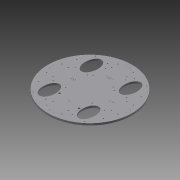
# Autodesk Inventor part: Base_Acryllic
Saved by Autodesk Inventor 2016 (Build 200138000, 138)
## iProperties
Created: 2016-03-29
Part Number: Base_Acryllic
Material: Generic
Document SubType Name: Modeling
Designer: Ethan
Density: 1 g/cm^3
Appearance: Default
Author: Ethan
Autodesk Inventor part; units mm, degrees
(part 1 of 2)
ref_plane "YZ Plane" through (0, 0, 0) normal (1, 0, 0) x (0, 1, 0)
ref_plane "XZ Plane" through (0, 0, 0) normal (0, 1, 0) x (-1, 0, 0)
ref_plane "XY Plane" through (0, 0, 0) normal (0, 0, 1) x (1, 0, 0)
sketch "Sketch1" plane through (0, 0, 0) normal (0, 1, 0) x (-1, 0, 0)
  circle A0 centre (0, 0) radius 139.7
  circle A1 centre (-118.5333, 25.4) radius 1.5875
  circle A2 centre (-97.3667, 25.4) radius 1.5875
  circle A3 centre (-118.5333, -25.4) radius 1.5875
  circle A4 centre (-97.3667, -25.4) radius 1.5875
  ellipse E0 centre (-65.0875, 69.8532) end of major axis (-65.0875, 36.5157) minor radius 20.6375
  ellipse E1 centre (-65.0875, -69.8532) end of major axis (-65.0875, -36.5157) minor radius 20.6375
  ellipse E2 centre (65.0875, 69.8532) end of major axis (65.0875, 36.5157) minor radius 20.6375
  ellipse E3 centre (65.0875, -69.8532) end of major axis (65.0875, -36.5157) minor radius 20.6375
  circle A5 centre (-38.1, 74.0494) radius 3.175
  circle A6 centre (38.1, 62.9369) radius 3.175
  circle A7 centre (85.725, 103.1907) radius 1.5875
  circle A8 centre (44.45, 103.1907) radius 1.5875
  circle A9 centre (85.725, 36.5157) radius 1.5875
  circle A10 centre (44.45, 36.5157) radius 1.5875
  circle A11 centre (44.45, -36.5157) radius 1.5875
  circle A12 centre (44.45, -103.1907) radius 1.5875
  circle A13 centre (85.725, -103.1907) radius 1.5875
  circle A14 centre (85.725, -36.5157) radius 1.5875
  circle A15 centre (33.3375, -43.706) radius 1.5875
  circle A16 centre (33.3375, -84.981) radius 1.5875
  circle A17 centre (-33.3375, -84.981) radius 1.5875
  circle A18 centre (-33.3375, -43.706) radius 1.5875
  circle A19 centre (-44.45, 36.5157) radius 1.5875
  circle A20 centre (-44.45, 103.1907) radius 1.5875
  circle A21 centre (-85.725, 103.1907) radius 1.5875
  circle A22 centre (-85.725, 36.5157) radius 1.5875
  circle A23 centre (-85.725, -36.5157) radius 1.5875
  circle A24 centre (-44.45, -36.5157) radius 1.5875
  circle A25 centre (-44.45, -103.1907) radius 1.5875
  circle A26 centre (-85.725, -103.1907) radius 1.5875
  circle A27 centre (-25.4, -118.5333) radius 1.5875
  circle A28 centre (-25.4, -97.3667) radius 1.5875
  circle A29 centre (25.4, -97.3667) radius 1.5875
  circle A30 centre (25.4, -118.5333) radius 1.5875
  circle A31 centre (118.5333, -25.4) radius 1.5875
  circle A32 centre (97.3667, -25.4) radius 1.5875
  circle A33 centre (97.3667, 25.4) radius 1.5875
  circle A34 centre (118.5333, 25.4) radius 1.5875
  circle A35 centre (25.4, 118.5333) radius 1.5875
  circle A36 centre (25.4, 97.3667) radius 1.5875
  circle A37 centre (-25.4, 97.3667) radius 1.5875
  circle A38 centre (-25.4, 118.5333) radius 1.5875
  circle A39 centre (107.2204, 62.9369) radius 1.5875
  circle A40 centre (-107.2204, 62.9369) radius 1.5875
  circle A41 centre (107.2204, -62.9369) radius 1.5875
  circle A42 centre (-107.2204, -62.9369) radius 1.5875
  circle A43 centre (6.25, 127) radius 1.1303
  circle A44 centre (-6.25, 127) radius 1.1303
  circle A45 centre (-127, 6.25) radius 1.1303
  circle A46 centre (-127, -6.25) radius 1.1303
  circle A47 centre (-6.25, -127) radius 1.1303
  circle A48 centre (6.25, -127) radius 1.1303
  circle A49 centre (127, -6.25) radius 1.1303
  circle A50 centre (127, 6.25) radius 1.1303
  line L0 (-37.9059, 73.7607) -> (38.0077, 73.7607) construction
  line L1 (38.0077, 73.7607) -> (38.0077, 62.868) construction
  line L2 (38.0077, 62.868) -> (-37.9059, 62.868) construction
  line L3 (-37.9059, 62.868) -> (-37.9059, 73.7607) construction
  line L4 (-34.0251, -43.002) -> (33.1245, -43.002) construction
  line L5 (33.1245, -43.002) -> (33.1245, -85.2103) construction
  line L6 (33.1245, -85.2103) -> (-34.0251, -85.2103) construction
  line L7 (-34.0251, -85.2103) -> (-34.0251, -43.002) construction
  line L8 (-12.7946, 24.5361) -> (126.9054, 24.5361) construction
  line L9 (126.9054, 24.5361) -> (126.9054, -26.2639) construction
  line L10 (126.9054, -26.2639) -> (-12.7946, -26.2639) construction
  line L11 (-12.7946, -26.2639) -> (-12.7946, 24.5361) construction
  line L12 (-126.5016, 32.6762) -> (-18.5516, 32.6762) construction
  line L13 (-18.5516, 32.6762) -> (-18.5516, -30.8238) construction
  line L14 (-18.5516, -30.8238) -> (-126.5016, -30.8238) construction
  line L15 (-126.5016, -30.8238) -> (-126.5016, 32.6762) construction
  line L16 (-6.9664, 66.7583) -> (-6.9664, 69.2258)
  line L17 (-6.9664, 69.2258) -> (-7.868, 69.2258)
  line L18 (-7.868, 69.2258) -> (-7.868, 69.8063)
  line L19 (-7.868, 69.8063) -> (-5.2991, 69.8063)
  line L20 (-5.2991, 69.8063) -> (-5.2991, 69.2258)
  line L21 (-5.2991, 69.2258) -> (-6.2007, 69.2258)
  line L22 (-6.2007, 69.2258) -> (-6.2007, 66.7583)
  line L23 (-6.2007, 66.7583) -> (-6.9664, 66.7583)
  line L24 (-3.7208, 67.8204) -> (-5.0768, 67.8204)
  line L25 (-5.0768, 67.8204) -> (-5.0768, 68.3885)
  line L26 (-5.0768, 68.3885) -> (-3.7208, 68.3885)
  line L27 (-3.7208, 68.3885) -> (-3.7208, 67.8204)
  spline S0 degree 2 poles (-0.742, 67.6919) (-0.742, 67.4647) (-0.9149, 67.1214) (-1.0581, 67.0078) knots 0 0 0 1 2 2 2
  spline S1 degree 2 poles (-1.0581, 67.0078) (-1.231, 66.8719) (-1.641, 66.7583) (-1.9597, 66.7583) knots 0 0 0 1 2 2 2
  line L28 (-1.9597, 66.7583) -> (-3.1774, 66.7583)
  line L29 (-3.1774, 66.7583) -> (-3.1774, 69.8063)
  line L30 (-3.1774, 69.8063) -> (-2.1029, 69.8063)
  spline S2 degree 2 poles (-2.1029, 69.8063) (-1.767, 69.8063) (-1.4212, 69.7544) (-1.2705, 69.6729) knots 0 0 0 1 2 2 2
  spline S3 degree 2 poles (-1.2705, 69.6729) (-1.1051, 69.5864) (-0.9445, 69.29) (-0.9445, 69.0974) knots 0 0 0 1 2 2 2
  spline S4 degree 2 poles (-0.9445, 69.0974) (-0.9445, 68.8751) (-1.1668, 68.5268) (-1.3644, 68.4453) knots 0 0 0 1 2 2 2
  line L31 (-1.3644, 68.4453) -> (-1.3644, 68.4305)
  spline S5 degree 2 poles (-1.3644, 68.4305) (-1.0804, 68.3712) (-0.742, 68.0032) (-0.742, 67.6919) knots 0 0 0 1 2 2 2
  spline S6 degree 2 poles (-1.5324, 67.7043) (-1.5324, 67.8476) (-1.646, 68.0081) (-1.7596, 68.0501) knots 0 0 0 1 2 2 2
  spline S7 degree 2 poles (-1.7596, 68.0501) (-1.8288, 68.0773) (-2.0733, 68.0822) (-2.2758, 68.0822) knots 0 0 0 1 2 2 2
  line L32 (-2.2758, 68.0822) -> (-2.4166, 68.0822)
  line L33 (-2.4166, 68.0822) -> (-2.4166, 67.314)
  line L34 (-2.4166, 67.314) -> (-2.3746, 67.314)
  spline S8 degree 2 poles (-2.3746, 67.314) (-2.0782, 67.314) (-1.851, 67.3214) (-1.7324, 67.3733) knots 0 0 0 1 2 2 2
  spline S9 degree 2 poles (-1.7324, 67.3733) (-1.6287, 67.4202) (-1.5324, 67.5931) (-1.5324, 67.7043) knots 0 0 0 1 2 2 2
  spline S10 degree 2 poles (-1.7226, 68.9467) (-1.7226, 69.0208) (-1.7991, 69.1764) (-1.8782, 69.211) knots 0 0 0 1 2 2 2
  spline S11 degree 2 poles (-1.8782, 69.211) (-1.9523, 69.2456) (-2.1598, 69.2505) (-2.3648, 69.2505) knots 0 0 0 1 2 2 2
  line L35 (-2.3648, 69.2505) -> (-2.4166, 69.2505)
  line L36 (-2.4166, 69.2505) -> (-2.4166, 68.6034)
  line L37 (-2.4166, 68.6034) -> (-2.3203, 68.6034)
  spline S12 degree 2 poles (-2.3203, 68.6034) (-2.1252, 68.6034) (-1.9671, 68.6108) (-1.8831, 68.6503) knots 0 0 0 1 2 2 2
  spline S13 degree 2 poles (-1.8831, 68.6503) (-1.7917, 68.6948) (-1.7226, 68.8454) (-1.7226, 68.9467) knots 0 0 0 1 2 2 2
  line L38 (0.372, 66.7583) -> (-0.3443, 66.7583)
  line L39 (-0.3443, 66.7583) -> (-0.3443, 69.9421)
  line L40 (-0.3443, 69.9421) -> (0.372, 69.9421)
  line L41 (0.372, 69.9421) -> (0.372, 66.7583)
  spline S14 degree 2 poles (3.1261, 67.9068) (3.1261, 67.3387) (2.5061, 66.6866) (1.9405, 66.6866) knots 0 0 0 1 2 2 2
  spline S15 degree 2 poles (1.9405, 66.6866) (1.3773, 66.6866) (0.7524, 67.3387) (0.7524, 67.9068) knots 0 0 0 1 2 2 2
  spline S16 degree 2 poles (0.7524, 67.9068) (0.7524, 68.4799) (1.3773, 69.1295) (1.9405, 69.1295) knots 0 0 0 1 2 2 2
  spline S17 degree 2 poles (1.9405, 69.1295) (2.5036, 69.1295) (3.1261, 68.4774) (3.1261, 67.9068) knots 0 0 0 1 2 2 2
  spline S18 degree 2 poles (2.3925, 67.9019) (2.3925, 68.1069) (2.3258, 68.3811) (2.2665, 68.4626) knots 0 0 0 1 2 2 2
  spline S19 degree 2 poles (2.2665, 68.4626) (2.2023, 68.549) (2.0417, 68.6157) (1.9405, 68.6157) knots 0 0 0 1 2 2 2
  spline S20 degree 2 poles (1.9405, 68.6157) (1.8417, 68.6157) (1.6861, 68.5565) (1.6218, 68.4725) knots 0 0 0 1 2 2 2
  spline S21 degree 2 poles (1.6218, 68.4725) (1.5601, 68.3934) (1.486, 68.1143) (1.486, 67.9019) knots 0 0 0 1 2 2 2
  spline S22 degree 2 poles (1.486, 67.9019) (1.486, 67.6919) (1.5552, 67.4326) (1.612, 67.3536) knots 0 0 0 1 2 2 2
  spline S23 degree 2 poles (1.612, 67.3536) (1.6688, 67.2745) (1.8417, 67.2004) (1.9454, 67.2004) knots 0 0 0 1 2 2 2
  spline S24 degree 2 poles (1.9454, 67.2004) (2.0319, 67.2004) (2.2097, 67.2745) (2.264, 67.3486) knots 0 0 0 1 2 2 2
  spline S25 degree 2 poles (2.264, 67.3486) (2.3258, 67.4351) (2.3925, 67.6845) (2.3925, 67.9019) knots 0 0 0 1 2 2 2
  spline S26 degree 2 poles (4.6328, 66.6965) (4.3487, 66.6965) (3.877, 66.8398) (3.7016, 66.988) knots 0 0 0 1 2 2 2
  spline S27 degree 2 poles (3.7016, 66.988) (3.5312, 67.1387) (3.3385, 67.5907) (3.3385, 67.897) knots 0 0 0 1 2 2 2
  spline S28 degree 2 poles (3.3385, 67.897) (3.3385, 68.2279) (3.546, 68.6898) (3.7263, 68.838) knots 0 0 0 1 2 2 2
  spline S29 degree 2 poles (3.7263, 68.838) (3.8967, 68.9813) (4.3611, 69.1196) (4.613, 69.1196) knots 0 0 0 1 2 2 2
  spline S30 degree 2 poles (4.613, 69.1196) (4.8032, 69.1196) (5.1836, 69.0307) (5.3763, 68.9344) knots 0 0 0 1 2 2 2
  line L42 (5.3763, 68.9344) -> (5.3763, 68.3218)
  line L43 (5.3763, 68.3218) -> (5.2849, 68.3218)
  spline S31 degree 2 poles (5.2849, 68.3218) (5.2404, 68.3638) (5.1169, 68.4626) (5.0428, 68.5021) knots 0 0 0 1 2 2 2
  spline S32 degree 2 poles (5.0428, 68.5021) (4.9638, 68.5466) (4.7686, 68.6059) (4.6476, 68.6059) knots 0 0 0 1 2 2 2
  spline S33 degree 2 poles (4.6476, 68.6059) (4.3734, 68.6059) (4.0721, 68.223) (4.0721, 67.897) knots 0 0 0 1 2 2 2
  spline S34 degree 2 poles (4.0721, 67.897) (4.0721, 67.5512) (4.3932, 67.2103) (4.66, 67.2103) knots 0 0 0 1 2 2 2
  spline S35 degree 2 poles (4.66, 67.2103) (4.7958, 67.2103) (4.9984, 67.272) (5.0725, 67.3165) knots 0 0 0 1 2 2 2
  spline S36 degree 2 poles (5.0725, 67.3165) (5.1441, 67.3585) (5.2478, 67.4524) (5.2849, 67.4894) knots 0 0 0 1 2 2 2
  line L44 (5.2849, 67.4894) -> (5.3763, 67.4894)
  line L45 (5.3763, 67.4894) -> (5.3763, 66.8744)
  spline S37 degree 2 poles (5.3763, 66.8744) (5.3145, 66.8472) (5.154, 66.778) (5.07, 66.7558) knots 0 0 0 1 2 2 2
  spline S38 degree 2 poles (5.07, 66.7558) (4.9662, 66.7262) (4.7835, 66.6965) (4.6328, 66.6965) knots 0 0 0 1 2 2 2
  line L46 (8.0192, 66.7583) -> (7.167, 66.7583)
  line L47 (7.167, 66.7583) -> (6.5446, 67.7562)
  line L48 (6.5446, 67.7562) -> (6.4334, 67.608)
  line L49 (6.4334, 67.608) -> (6.4334, 66.7583)
  line L50 (6.4334, 66.7583) -> (5.7171, 66.7583)
  line L51 (5.7171, 66.7583) -> (5.7171, 69.9421)
  line L52 (5.7171, 69.9421) -> (6.4334, 69.9421)
  line L53 (6.4334, 69.9421) -> (6.4334, 68.1588)
  line L54 (6.4334, 68.1588) -> (7.1127, 69.0579)
  line L55 (7.1127, 69.0579) -> (7.9599, 69.0579)
  line L56 (7.9599, 69.0579) -> (7.1547, 68.0674)
  line L57 (7.1547, 68.0674) -> (8.0192, 66.7583)
  line L58 (51.3892, 2.9174) -> (50.0875, 0.4746)
  line L59 (50.0875, 0.4746) -> (49.2378, 0.4746)
  line L60 (49.2378, 0.4746) -> (50.5987, 2.947)
  line L61 (50.5987, 2.947) -> (49.1464, 2.947)
  line L62 (49.1464, 2.947) -> (49.1464, 3.5226)
  line L63 (49.1464, 3.5226) -> (51.3892, 3.5226)
  line L64 (51.3892, 3.5226) -> (51.3892, 2.9174)
  line L65 (52.5921, 0.4746) -> (51.8683, 0.4746)
  line L66 (51.8683, 0.4746) -> (51.8683, 1.2798)
  line L67 (51.8683, 1.2798) -> (52.5921, 1.2798)
  line L68 (52.5921, 1.2798) -> (52.5921, 0.4746)
  line L69 (55.435, 0.4746) -> (53.1947, 0.4746)
  line L70 (53.1947, 0.4746) -> (53.1947, 0.971)
  spline S39 degree 2 poles (53.1947, 0.971) (53.4788, 1.1983) (53.9333, 1.5984) (54.1037, 1.7787) knots 0 0 0 1 2 2 2
  spline S40 degree 2 poles (54.1037, 1.7787) (54.3285, 2.0134) (54.5285, 2.3715) (54.5285, 2.5592) knots 0 0 0 1 2 2 2
  spline S41 degree 2 poles (54.5285, 2.5592) (54.5285, 2.7717) (54.2741, 2.9989) (54.0469, 2.9989) knots 0 0 0 1 2 2 2
  spline S42 degree 2 poles (54.0469, 2.9989) (53.9308, 2.9989) (53.7233, 2.9421) (53.6171, 2.8976) knots 0 0 0 1 2 2 2
  spline S43 degree 2 poles (53.6171, 2.8976) (53.5134, 2.8507) (53.3652, 2.7519) (53.3281, 2.7272) knots 0 0 0 1 2 2 2
  line L71 (53.3281, 2.7272) -> (53.2688, 2.7272)
  line L72 (53.2688, 2.7272) -> (53.2688, 3.3916)
  spline S44 degree 2 poles (53.2688, 3.3916) (53.3973, 3.4534) (53.9456, 3.5818) (54.2, 3.5818) knots 0 0 0 1 2 2 2
  spline S45 degree 2 poles (54.2, 3.5818) (54.7434, 3.5818) (55.3017, 3.0977) (55.3017, 2.6605) knots 0 0 0 1 2 2 2
  spline S46 degree 2 poles (55.3017, 2.6605) (55.3017, 2.3913) (55.0472, 1.8726) (54.7533, 1.5762) knots 0 0 0 1 2 2 2
  spline S47 degree 2 poles (54.7533, 1.5762) (54.5681, 1.3934) (54.2198, 1.1093) (54.1432, 1.0501) knots 0 0 0 1 2 2 2
  line L73 (54.1432, 1.0501) -> (55.435, 1.0501)
  line L74 (55.435, 1.0501) -> (55.435, 0.4746)
  line L75 (59.6439, 3.5226) -> (58.5967, 0.4746)
  line L76 (58.5967, 0.4746) -> (57.7988, 0.4746)
  line L77 (57.7988, 0.4746) -> (56.7516, 3.5226)
  line L78 (56.7516, 3.5226) -> (57.5444, 3.5226)
  line L79 (57.5444, 3.5226) -> (58.2089, 1.4551)
  line L80 (58.2089, 1.4551) -> (58.8708, 3.5226)
  line L81 (58.8708, 3.5226) -> (59.6439, 3.5226)
  spline S48 degree 2 poles (62.0917, 1.6231) (62.0917, 1.055) (61.4718, 0.4029) (60.9061, 0.4029) knots 0 0 0 1 2 2 2
  spline S49 degree 2 poles (60.9061, 0.4029) (60.343, 0.4029) (59.718, 1.055) (59.718, 1.6231) knots 0 0 0 1 2 2 2
  spline S50 degree 2 poles (59.718, 1.6231) (59.718, 2.1962) (60.343, 2.8458) (60.9061, 2.8458) knots 0 0 0 1 2 2 2
  spline S51 degree 2 poles (60.9061, 2.8458) (61.4693, 2.8458) (62.0917, 2.1937) (62.0917, 1.6231) knots 0 0 0 1 2 2 2
  spline S52 degree 2 poles (61.3581, 1.6182) (61.3581, 1.8232) (61.2914, 2.0974) (61.2322, 2.1789) knots 0 0 0 1 2 2 2
  spline S53 degree 2 poles (61.2322, 2.1789) (61.1679, 2.2653) (61.0074, 2.332) (60.9061, 2.332) knots 0 0 0 1 2 2 2
  spline S54 degree 2 poles (60.9061, 2.332) (60.8073, 2.332) (60.6517, 2.2727) (60.5875, 2.1887) knots 0 0 0 1 2 2 2
  spline S55 degree 2 poles (60.5875, 2.1887) (60.5257, 2.1097) (60.4516, 1.8306) (60.4516, 1.6182) knots 0 0 0 1 2 2 2
  spline S56 degree 2 poles (60.4516, 1.6182) (60.4516, 1.4082) (60.5208, 1.1489) (60.5776, 1.0698) knots 0 0 0 1 2 2 2
  spline S57 degree 2 poles (60.5776, 1.0698) (60.6344, 0.9908) (60.8073, 0.9167) (60.9111, 0.9167) knots 0 0 0 1 2 2 2
  spline S58 degree 2 poles (60.9111, 0.9167) (60.9975, 0.9167) (61.1754, 0.9908) (61.2297, 1.0649) knots 0 0 0 1 2 2 2
  spline S59 degree 2 poles (61.2297, 1.0649) (61.2914, 1.1513) (61.3581, 1.4008) (61.3581, 1.6182) knots 0 0 0 1 2 2 2
  line L82 (63.1884, 0.4746) -> (62.4721, 0.4746)
  line L83 (62.4721, 0.4746) -> (62.4721, 3.6584)
  line L84 (62.4721, 3.6584) -> (63.1884, 3.6584)
  line L85 (63.1884, 3.6584) -> (63.1884, 0.4746)
  spline S60 degree 2 poles (64.6161, 0.4301) (64.1789, 0.4301) (63.7788, 0.7907) (63.7788, 1.2007) knots 0 0 0 1 2 2 2
  line L86 (63.7788, 1.2007) -> (63.7788, 2.2752)
  line L87 (63.7788, 2.2752) -> (63.5046, 2.2752)
  line L88 (63.5046, 2.2752) -> (63.5046, 2.7741)
  line L89 (63.5046, 2.7741) -> (63.7788, 2.7741)
  line L90 (63.7788, 2.7741) -> (63.7788, 3.4312)
  line L91 (63.7788, 3.4312) -> (64.4951, 3.4312)
  line L92 (64.4951, 3.4312) -> (64.4951, 2.7741)
  line L93 (64.4951, 2.7741) -> (65.1867, 2.7741)
  line L94 (65.1867, 2.7741) -> (65.1867, 2.2752)
  line L95 (65.1867, 2.2752) -> (64.4951, 2.2752)
  line L96 (64.4951, 2.2752) -> (64.4951, 1.4576)
  spline S61 degree 2 poles (64.4951, 1.4576) (64.4951, 1.3366) (64.5, 1.1563) (64.5296, 1.0846) knots 0 0 0 1 2 2 2
  spline S62 degree 2 poles (64.5296, 1.0846) (64.5593, 1.013) (64.705, 0.929) (64.8433, 0.929) knots 0 0 0 1 2 2 2
  spline S63 degree 2 poles (64.8433, 0.929) (64.9026, 0.929) (65.0879, 0.9784) (65.1249, 0.9982) knots 0 0 0 1 2 2 2
  line L97 (65.1249, 0.9982) -> (65.1867, 0.9982)
  line L98 (65.1867, 0.9982) -> (65.1867, 0.4943)
  spline S64 degree 2 poles (65.1867, 0.4943) (65.0706, 0.4647) (64.8088, 0.4301) (64.6161, 0.4301) knots 0 0 0 1 2 2 2
  spline S65 degree 2 poles (52.0079, -3.6102) (52.0079, -3.8375) (51.835, -4.1808) (51.6917, -4.2944) knots 0 0 0 1 2 2 2
  spline S66 degree 2 poles (51.6917, -4.2944) (51.5188, -4.4303) (51.1088, -4.5439) (50.7902, -4.5439) knots 0 0 0 1 2 2 2
  line L99 (50.7902, -4.5439) -> (49.5725, -4.5439)
  line L100 (49.5725, -4.5439) -> (49.5725, -1.4959)
  line L101 (49.5725, -1.4959) -> (50.6469, -1.4959)
  spline S67 degree 2 poles (50.6469, -1.4959) (50.9828, -1.4959) (51.3286, -1.5478) (51.4793, -1.6293) knots 0 0 0 1 2 2 2
  spline S68 degree 2 poles (51.4793, -1.6293) (51.6448, -1.7157) (51.8054, -2.0121) (51.8054, -2.2048) knots 0 0 0 1 2 2 2
  spline S69 degree 2 poles (51.8054, -2.2048) (51.8054, -2.4271) (51.583, -2.7754) (51.3854, -2.8569) knots 0 0 0 1 2 2 2
  line L102 (51.3854, -2.8569) -> (51.3854, -2.8717)
  spline S70 degree 2 poles (51.3854, -2.8717) (51.6695, -2.931) (52.0079, -3.299) (52.0079, -3.6102) knots 0 0 0 1 2 2 2
  spline S71 degree 2 poles (51.2175, -3.5979) (51.2175, -3.4546) (51.1039, -3.2941) (50.9902, -3.2521) knots 0 0 0 1 2 2 2
  spline S72 degree 2 poles (50.9902, -3.2521) (50.9211, -3.2249) (50.6766, -3.22) (50.474, -3.22) knots 0 0 0 1 2 2 2
  line L103 (50.474, -3.22) -> (50.3332, -3.22)
  line L104 (50.3332, -3.22) -> (50.3332, -3.9881)
  line L105 (50.3332, -3.9881) -> (50.3752, -3.9881)
  spline S73 degree 2 poles (50.3752, -3.9881) (50.6716, -3.9881) (50.8989, -3.9807) (51.0174, -3.9289) knots 0 0 0 1 2 2 2
  spline S74 degree 2 poles (51.0174, -3.9289) (51.1212, -3.8819) (51.2175, -3.709) (51.2175, -3.5979) knots 0 0 0 1 2 2 2
  spline S75 degree 2 poles (51.0273, -2.3555) (51.0273, -2.2814) (50.9507, -2.1258) (50.8717, -2.0912) knots 0 0 0 1 2 2 2
  spline S76 degree 2 poles (50.8717, -2.0912) (50.7976, -2.0566) (50.5901, -2.0517) (50.3851, -2.0517) knots 0 0 0 1 2 2 2
  line L106 (50.3851, -2.0517) -> (50.3332, -2.0517)
  line L107 (50.3332, -2.0517) -> (50.3332, -2.6988)
  line L108 (50.3332, -2.6988) -> (50.4296, -2.6988)
  spline S77 degree 2 poles (50.4296, -2.6988) (50.6247, -2.6988) (50.7828, -2.6914) (50.8667, -2.6519) knots 0 0 0 1 2 2 2
  spline S78 degree 2 poles (50.8667, -2.6519) (50.9581, -2.6074) (51.0273, -2.4567) (51.0273, -2.3555) knots 0 0 0 1 2 2 2
  spline S79 degree 2 poles (53.6727, -4.2994) (53.5986, -4.3611) (53.4825, -4.4599) (53.3837, -4.5093) knots 0 0 0 1 2 2 2
  spline S80 degree 2 poles (53.3837, -4.5093) (53.2874, -4.5563) (53.1046, -4.6057) (52.9416, -4.6057) knots 0 0 0 1 2 2 2
  spline S81 degree 2 poles (52.9416, -4.6057) (52.6353, -4.6057) (52.2327, -4.1956) (52.2327, -3.8844) knots 0 0 0 1 2 2 2
  spline S82 degree 2 poles (52.2327, -3.8844) (52.2327, -3.63) (52.4377, -3.3138) (52.6303, -3.2224) knots 0 0 0 1 2 2 2
  spline S83 degree 2 poles (52.6303, -3.2224) (52.8255, -3.1286) (53.3664, -3.0545) (53.6776, -3.0347) knots 0 0 0 1 2 2 2
  line L109 (53.6776, -3.0347) -> (53.6776, -3.0224)
  spline S84 degree 2 poles (53.6776, -3.0224) (53.6776, -2.8322) (53.396, -2.6864) (53.1145, -2.6864) knots 0 0 0 1 2 2 2
  spline S85 degree 2 poles (53.1145, -2.6864) (52.9885, -2.6864) (52.6476, -2.7778) (52.4871, -2.8495) knots 0 0 0 1 2 2 2
  line L110 (52.4871, -2.8495) -> (52.4253, -2.8495)
  line L111 (52.4253, -2.8495) -> (52.4253, -2.2937)
  spline S86 degree 2 poles (52.4253, -2.2937) (52.5315, -2.2641) (53.0058, -2.1801) (53.2478, -2.1801) knots 0 0 0 1 2 2 2
  spline S87 degree 2 poles (53.2478, -2.1801) (53.8406, -2.1801) (54.384, -2.5753) (54.384, -2.9804) knots 0 0 0 1 2 2 2
  line L112 (54.384, -2.9804) -> (54.384, -4.5439)
  line L113 (54.384, -4.5439) -> (53.6727, -4.5439)
  line L114 (53.6727, -4.5439) -> (53.6727, -4.2994)
  line L115 (53.6727, -3.9437) -> (53.6727, -3.467)
  spline S88 degree 2 poles (53.6727, -3.467) (53.4899, -3.4843) (53.2651, -3.5114) (53.1564, -3.551) knots 0 0 0 1 2 2 2
  spline S89 degree 2 poles (53.1564, -3.551) (53.0601, -3.5831) (52.9564, -3.7164) (52.9564, -3.8251) knots 0 0 0 1 2 2 2
  spline S90 degree 2 poles (52.9564, -3.8251) (52.9564, -3.9857) (53.1317, -4.1067) (53.3022, -4.1067) knots 0 0 0 1 2 2 2
  spline S91 degree 2 poles (53.3022, -4.1067) (53.396, -4.1067) (53.5936, -4.0203) (53.6727, -3.9437) knots 0 0 0 1 2 2 2
  spline S92 degree 2 poles (55.7944, -4.5884) (55.3572, -4.5884) (54.9571, -4.2277) (54.9571, -3.8177) knots 0 0 0 1 2 2 2
  line L116 (54.9571, -3.8177) -> (54.9571, -2.7433)
  line L117 (54.9571, -2.7433) -> (54.6829, -2.7433)
  line L118 (54.6829, -2.7433) -> (54.6829, -2.2443)
  line L119 (54.6829, -2.2443) -> (54.9571, -2.2443)
  line L120 (54.9571, -2.2443) -> (54.9571, -1.5873)
  line L121 (54.9571, -1.5873) -> (55.6734, -1.5873)
  line L122 (55.6734, -1.5873) -> (55.6734, -2.2443)
  line L123 (55.6734, -2.2443) -> (56.365, -2.2443)
  line L124 (56.365, -2.2443) -> (56.365, -2.7433)
  line L125 (56.365, -2.7433) -> (55.6734, -2.7433)
  line L126 (55.6734, -2.7433) -> (55.6734, -3.5608)
  spline S93 degree 2 poles (55.6734, -3.5608) (55.6734, -3.6819) (55.6783, -3.8622) (55.708, -3.9338) knots 0 0 0 1 2 2 2
  spline S94 degree 2 poles (55.708, -3.9338) (55.7376, -4.0054) (55.8833, -4.0894) (56.0217, -4.0894) knots 0 0 0 1 2 2 2
  spline S95 degree 2 poles (56.0217, -4.0894) (56.0809, -4.0894) (56.2662, -4.04) (56.3033, -4.0203) knots 0 0 0 1 2 2 2
  line L127 (56.3033, -4.0203) -> (56.365, -4.0203)
  line L128 (56.365, -4.0203) -> (56.365, -4.5241)
  spline S96 degree 2 poles (56.365, -4.5241) (56.2489, -4.5538) (55.9871, -4.5884) (55.7944, -4.5884) knots 0 0 0 1 2 2 2
  spline S97 degree 2 poles (57.5358, -4.5884) (57.0986, -4.5884) (56.6985, -4.2277) (56.6985, -3.8177) knots 0 0 0 1 2 2 2
  line L129 (56.6985, -3.8177) -> (56.6985, -2.7433)
  line L130 (56.6985, -2.7433) -> (56.4243, -2.7433)
  line L131 (56.4243, -2.7433) -> (56.4243, -2.2443)
  line L132 (56.4243, -2.2443) -> (56.6985, -2.2443)
  line L133 (56.6985, -2.2443) -> (56.6985, -1.5873)
  line L134 (56.6985, -1.5873) -> (57.4148, -1.5873)
  line L135 (57.4148, -1.5873) -> (57.4148, -2.2443)
  line L136 (57.4148, -2.2443) -> (58.1064, -2.2443)
  line L137 (58.1064, -2.2443) -> (58.1064, -2.7433)
  line L138 (58.1064, -2.7433) -> (57.4148, -2.7433)
  line L139 (57.4148, -2.7433) -> (57.4148, -3.5608)
  spline S98 degree 2 poles (57.4148, -3.5608) (57.4148, -3.6819) (57.4197, -3.8622) (57.4493, -3.9338) knots 0 0 0 1 2 2 2
  spline S99 degree 2 poles (57.4493, -3.9338) (57.479, -4.0054) (57.6247, -4.0894) (57.763, -4.0894) knots 0 0 0 1 2 2 2
  spline S100 degree 2 poles (57.763, -4.0894) (57.8223, -4.0894) (58.0076, -4.04) (58.0446, -4.0203) knots 0 0 0 1 2 2 2
  line L140 (58.0446, -4.0203) -> (58.1064, -4.0203)
  line L141 (58.1064, -4.0203) -> (58.1064, -4.5241)
  spline S101 degree 2 poles (58.1064, -4.5241) (57.9903, -4.5538) (57.7284, -4.5884) (57.5358, -4.5884) knots 0 0 0 1 2 2 2
  spline S102 degree 2 poles (59.576, -4.6057) (58.9239, -4.6057) (58.2299, -3.9832) (58.2299, -3.4077) knots 0 0 0 1 2 2 2
  spline S103 degree 2 poles (58.2299, -3.4077) (58.2299, -2.8445) (58.877, -2.1727) (59.4599, -2.1727) knots 0 0 0 1 2 2 2
  spline S104 degree 2 poles (59.4599, -2.1727) (59.986, -2.1727) (60.5196, -2.7433) (60.5196, -3.2718) knots 0 0 0 1 2 2 2
  line L142 (60.5196, -3.2718) -> (60.5196, -3.5312)
  line L143 (60.5196, -3.5312) -> (58.9462, -3.5312)
  spline S105 degree 2 poles (58.9462, -3.5312) (58.956, -3.6917) (59.0721, -3.9042) (59.166, -3.9684) knots 0 0 0 1 2 2 2
  spline S106 degree 2 poles (59.166, -3.9684) (59.2574, -4.0326) (59.5044, -4.0869) (59.6501, -4.0869) knots 0 0 0 1 2 2 2
  spline S107 degree 2 poles (59.6501, -4.0869) (59.7736, -4.0869) (60.0157, -4.0326) (60.117, -3.9857) knots 0 0 0 1 2 2 2
  spline S108 degree 2 poles (60.117, -3.9857) (60.2059, -3.9486) (60.3541, -3.8572) (60.401, -3.8227) knots 0 0 0 1 2 2 2
  line L144 (60.401, -3.8227) -> (60.4776, -3.8227)
  line L145 (60.4776, -3.8227) -> (60.4776, -4.4155)
  spline S109 degree 2 poles (60.4776, -4.4155) (60.3887, -4.45) (60.2454, -4.5093) (60.117, -4.539) knots 0 0 0 1 2 2 2
  spline S110 degree 2 poles (60.117, -4.539) (60.0009, -4.5711) (59.7539, -4.6057) (59.576, -4.6057) knots 0 0 0 1 2 2 2
  spline S111 degree 2 poles (59.8131, -3.0989) (59.8082, -2.8717) (59.6081, -2.6321) (59.4031, -2.6321) knots 0 0 0 1 2 2 2
  spline S112 degree 2 poles (59.4031, -2.6321) (59.1932, -2.6321) (58.956, -2.884) (58.9437, -3.0989) knots 0 0 0 1 2 2 2
  line L146 (58.9437, -3.0989) -> (59.8131, -3.0989)
  line L147 (62.4314, -2.9236) -> (62.3721, -2.9236)
  spline S113 degree 2 poles (62.3721, -2.9236) (62.3301, -2.9088) (62.1745, -2.8939) (62.0806, -2.8939) knots 0 0 0 1 2 2 2
  spline S114 degree 2 poles (62.0806, -2.8939) (61.9695, -2.8939) (61.72, -2.9606) (61.6039, -3.0051) knots 0 0 0 1 2 2 2
  line L148 (61.6039, -3.0051) -> (61.6039, -4.5439)
  line L149 (61.6039, -4.5439) -> (60.8876, -4.5439)
  line L150 (60.8876, -4.5439) -> (60.8876, -2.2443)
  line L151 (60.8876, -2.2443) -> (61.6039, -2.2443)
  line L152 (61.6039, -2.2443) -> (61.6039, -2.5753)
  spline S115 degree 2 poles (61.6039, -2.5753) (61.6533, -2.5308) (61.8262, -2.3925) (61.8978, -2.3505) knots 0 0 0 1 2 2 2
  spline S116 degree 2 poles (61.8978, -2.3505) (61.9769, -2.3036) (62.1844, -2.2369) (62.2757, -2.2369) knots 0 0 0 1 2 2 2
  spline S117 degree 2 poles (62.2757, -2.2369) (62.3103, -2.2369) (62.3968, -2.2418) (62.4314, -2.2443) knots 0 0 0 1 2 2 2
  line L153 (62.4314, -2.2443) -> (62.4314, -2.9236)
  line L154 (64.8495, -2.2443) -> (63.6911, -5.3862)
  line L155 (63.6911, -5.3862) -> (62.9204, -5.3862)
  line L156 (62.9204, -5.3862) -> (63.2687, -4.4871)
  line L157 (63.2687, -4.4871) -> (62.4264, -2.2443)
  line L158 (62.4264, -2.2443) -> (63.1773, -2.2443)
  line L159 (63.1773, -2.2443) -> (63.6614, -3.6868)
  line L160 (63.6614, -3.6868) -> (64.1134, -2.2443)
  line L161 (64.1134, -2.2443) -> (64.8495, -2.2443)
  line L162 (-5.6188, -59.7086) -> (-6.6661, -62.7566)
  line L163 (-6.6661, -62.7566) -> (-7.4639, -62.7566)
  line L164 (-7.4639, -62.7566) -> (-8.5112, -59.7086)
  line L165 (-8.5112, -59.7086) -> (-7.7183, -59.7086)
  line L166 (-7.7183, -59.7086) -> (-7.0539, -61.776)
  line L167 (-7.0539, -61.776) -> (-6.3919, -59.7086)
  line L168 (-6.3919, -59.7086) -> (-5.6188, -59.7086)
  spline S118 degree 2 poles (-3.171, -61.608) (-3.171, -62.1761) (-3.791, -62.8282) (-4.3566, -62.8282) knots 0 0 0 1 2 2 2
  spline S119 degree 2 poles (-4.3566, -62.8282) (-4.9198, -62.8282) (-5.5447, -62.1761) (-5.5447, -61.608) knots 0 0 0 1 2 2 2
  spline S120 degree 2 poles (-5.5447, -61.608) (-5.5447, -61.035) (-4.9198, -60.3854) (-4.3566, -60.3854) knots 0 0 0 1 2 2 2
  spline S121 degree 2 poles (-4.3566, -60.3854) (-3.7935, -60.3854) (-3.171, -61.0374) (-3.171, -61.608) knots 0 0 0 1 2 2 2
  spline S122 degree 2 poles (-3.9046, -61.613) (-3.9046, -61.4079) (-3.9713, -61.1338) (-4.0306, -61.0523) knots 0 0 0 1 2 2 2
  spline S123 degree 2 poles (-4.0306, -61.0523) (-4.0948, -60.9658) (-4.2554, -60.8991) (-4.3566, -60.8991) knots 0 0 0 1 2 2 2
  spline S124 degree 2 poles (-4.3566, -60.8991) (-4.4554, -60.8991) (-4.611, -60.9584) (-4.6753, -61.0424) knots 0 0 0 1 2 2 2
  spline S125 degree 2 poles (-4.6753, -61.0424) (-4.737, -61.1214) (-4.8111, -61.4005) (-4.8111, -61.613) knots 0 0 0 1 2 2 2
  spline S126 degree 2 poles (-4.8111, -61.613) (-4.8111, -61.8229) (-4.7419, -62.0823) (-4.6851, -62.1613) knots 0 0 0 1 2 2 2
  spline S127 degree 2 poles (-4.6851, -62.1613) (-4.6283, -62.2403) (-4.4554, -62.3144) (-4.3517, -62.3144) knots 0 0 0 1 2 2 2
  spline S128 degree 2 poles (-4.3517, -62.3144) (-4.2652, -62.3144) (-4.0874, -62.2403) (-4.0331, -62.1662) knots 0 0 0 1 2 2 2
  spline S129 degree 2 poles (-4.0331, -62.1662) (-3.9713, -62.0798) (-3.9046, -61.8303) (-3.9046, -61.613) knots 0 0 0 1 2 2 2
  line L169 (-2.0743, -62.7566) -> (-2.7906, -62.7566)
  line L170 (-2.7906, -62.7566) -> (-2.7906, -59.5727)
  line L171 (-2.7906, -59.5727) -> (-2.0743, -59.5727)
  line L172 (-2.0743, -59.5727) -> (-2.0743, -62.7566)
  spline S130 degree 2 poles (-0.6467, -62.801) (-1.0839, -62.801) (-1.484, -62.4404) (-1.484, -62.0304) knots 0 0 0 1 2 2 2
  line L173 (-1.484, -62.0304) -> (-1.484, -60.9559)
  line L174 (-1.484, -60.9559) -> (-1.7582, -60.9559)
  line L175 (-1.7582, -60.9559) -> (-1.7582, -60.457)
  line L176 (-1.7582, -60.457) -> (-1.484, -60.457)
  line L177 (-1.484, -60.457) -> (-1.484, -59.8)
  line L178 (-1.484, -59.8) -> (-0.7677, -59.8)
  line L179 (-0.7677, -59.8) -> (-0.7677, -60.457)
  line L180 (-0.7677, -60.457) -> (-0.0761, -60.457)
  line L181 (-0.0761, -60.457) -> (-0.0761, -60.9559)
  line L182 (-0.0761, -60.9559) -> (-0.7677, -60.9559)
  line L183 (-0.7677, -60.9559) -> (-0.7677, -61.7735)
  spline S131 degree 2 poles (-0.7677, -61.7735) (-0.7677, -61.8945) (-0.7628, -62.0749) (-0.7331, -62.1465) knots 0 0 0 1 2 2 2
  spline S132 degree 2 poles (-0.7331, -62.1465) (-0.7035, -62.2181) (-0.5577, -62.3021) (-0.4194, -62.3021) knots 0 0 0 1 2 2 2
  spline S133 degree 2 poles (-0.4194, -62.3021) (-0.3601, -62.3021) (-0.1749, -62.2527) (-0.1378, -62.2329) knots 0 0 0 1 2 2 2
  line L184 (-0.1378, -62.2329) -> (-0.0761, -62.2329)
  line L185 (-0.0761, -62.2329) -> (-0.0761, -62.7368)
  spline S134 degree 2 poles (-0.0761, -62.7368) (-0.1922, -62.7665) (-0.454, -62.801) (-0.6467, -62.801) knots 0 0 0 1 2 2 2
  spline S135 degree 2 poles (1.4825, -62.512) (1.4084, -62.5738) (1.2923, -62.6726) (1.1935, -62.722) knots 0 0 0 1 2 2 2
  spline S136 degree 2 poles (1.1935, -62.722) (1.0972, -62.7689) (0.9144, -62.8183) (0.7514, -62.8183) knots 0 0 0 1 2 2 2
  spline S137 degree 2 poles (0.7514, -62.8183) (0.4451, -62.8183) (0.0425, -62.4083) (0.0425, -62.0971) knots 0 0 0 1 2 2 2
  spline S138 degree 2 poles (0.0425, -62.0971) (0.0425, -61.8427) (0.2475, -61.5265) (0.4401, -61.4351) knots 0 0 0 1 2 2 2
  spline S139 degree 2 poles (0.4401, -61.4351) (0.6353, -61.3413) (1.1762, -61.2672) (1.4874, -61.2474) knots 0 0 0 1 2 2 2
  line L186 (1.4874, -61.2474) -> (1.4874, -61.235)
  spline S140 degree 2 poles (1.4874, -61.235) (1.4874, -61.0449) (1.2059, -60.8991) (0.9243, -60.8991) knots 0 0 0 1 2 2 2
  spline S141 degree 2 poles (0.9243, -60.8991) (0.7983, -60.8991) (0.4574, -60.9905) (0.2969, -61.0621) knots 0 0 0 1 2 2 2
  line L187 (0.2969, -61.0621) -> (0.2351, -61.0621)
  line L188 (0.2351, -61.0621) -> (0.2351, -60.5064)
  spline S142 degree 2 poles (0.2351, -60.5064) (0.3413, -60.4768) (0.8156, -60.3928) (1.0577, -60.3928) knots 0 0 0 1 2 2 2
  spline S143 degree 2 poles (1.0577, -60.3928) (1.6505, -60.3928) (2.1939, -60.788) (2.1939, -61.1931) knots 0 0 0 1 2 2 2
  line L189 (2.1939, -61.1931) -> (2.1939, -62.7566)
  line L190 (2.1939, -62.7566) -> (1.4825, -62.7566)
  line L191 (1.4825, -62.7566) -> (1.4825, -62.512)
  line L192 (1.4825, -62.1564) -> (1.4825, -61.6796)
  spline S144 degree 2 poles (1.4825, -61.6796) (1.2997, -61.6969) (1.0749, -61.7241) (0.9663, -61.7636) knots 0 0 0 1 2 2 2
  spline S145 degree 2 poles (0.9663, -61.7636) (0.8699, -61.7957) (0.7662, -61.9291) (0.7662, -62.0378) knots 0 0 0 1 2 2 2
  spline S146 degree 2 poles (0.7662, -62.0378) (0.7662, -62.1984) (0.9416, -62.3194) (1.112, -62.3194) knots 0 0 0 1 2 2 2
  spline S147 degree 2 poles (1.112, -62.3194) (1.2059, -62.3194) (1.4035, -62.2329) (1.4825, -62.1564) knots 0 0 0 1 2 2 2
  spline S148 degree 2 poles (4.8145, -62.4923) (4.8145, -62.8109) (4.6293, -63.258) (4.4712, -63.3815) knots 0 0 0 1 2 2 2
  spline S149 degree 2 poles (4.4712, -63.3815) (4.3107, -63.5075) (3.8661, -63.6211) (3.5944, -63.6211) knots 0 0 0 1 2 2 2
  spline S150 degree 2 poles (3.5944, -63.6211) (3.3646, -63.6211) (2.9522, -63.5618) (2.8015, -63.5223) knots 0 0 0 1 2 2 2
  line L193 (2.8015, -63.5223) -> (2.8015, -62.9468)
  line L194 (2.8015, -62.9468) -> (2.8855, -62.9468)
  spline S151 degree 2 poles (2.8855, -62.9468) (2.9373, -62.9665) (3.0831, -63.0159) (3.1572, -63.0357) knots 0 0 0 1 2 2 2
  spline S152 degree 2 poles (3.1572, -63.0357) (3.2461, -63.0579) (3.414, -63.0876) (3.5005, -63.0876) knots 0 0 0 1 2 2 2
  spline S153 degree 2 poles (3.5005, -63.0876) (3.6833, -63.0876) (3.9253, -63.0135) (3.9871, -62.9443) knots 0 0 0 1 2 2 2
  spline S154 degree 2 poles (3.9871, -62.9443) (4.0488, -62.8727) (4.0982, -62.68) (4.0982, -62.5318) knots 0 0 0 1 2 2 2
  line L195 (4.0982, -62.5318) -> (4.0982, -62.4898)
  spline S155 degree 2 poles (4.0982, -62.4898) (3.9772, -62.596) (3.661, -62.7245) (3.4931, -62.7245) knots 0 0 0 1 2 2 2
  spline S156 degree 2 poles (3.4931, -62.7245) (3.046, -62.7245) (2.5619, -62.144) (2.5619, -61.5487) knots 0 0 0 1 2 2 2
  spline S157 degree 2 poles (2.5619, -61.5487) (2.5619, -61.2795) (2.7101, -60.8497) (2.8435, -60.6991) knots 0 0 0 1 2 2 2
  spline S158 degree 2 poles (2.8435, -60.6991) (2.9719, -60.5533) (3.3301, -60.3952) (3.5252, -60.3952) knots 0 0 0 1 2 2 2
  spline S159 degree 2 poles (3.5252, -60.3952) (3.7006, -60.3952) (3.9797, -60.4842) (4.0933, -60.5583) knots 0 0 0 1 2 2 2
  line L196 (4.0933, -60.5583) -> (4.1205, -60.457)
  line L197 (4.1205, -60.457) -> (4.8145, -60.457)
  line L198 (4.8145, -60.457) -> (4.8145, -62.4923)
  line L199 (4.0982, -62.0329) -> (4.0982, -60.9905)
  spline S160 degree 2 poles (4.0982, -60.9905) (4.0464, -60.9658) (3.8908, -60.9337) (3.8117, -60.9337) knots 0 0 0 1 2 2 2
  spline S161 degree 2 poles (3.8117, -60.9337) (3.5548, -60.9337) (3.2955, -61.2672) (3.2955, -61.566) knots 0 0 0 1 2 2 2
  spline S162 degree 2 poles (3.2955, -61.566) (3.2955, -61.7142) (3.335, -61.9217) (3.3869, -62.0008) knots 0 0 0 1 2 2 2
  spline S163 degree 2 poles (3.3869, -62.0008) (3.4387, -62.0798) (3.6042, -62.1588) (3.7327, -62.1588) knots 0 0 0 1 2 2 2
  spline S164 degree 2 poles (3.7327, -62.1588) (3.829, -62.1588) (4.0143, -62.0921) (4.0982, -62.0329) knots 0 0 0 1 2 2 2
  spline S165 degree 2 poles (6.5411, -62.8183) (5.889, -62.8183) (5.1949, -62.1959) (5.1949, -61.6204) knots 0 0 0 1 2 2 2
  spline S166 degree 2 poles (5.1949, -61.6204) (5.1949, -61.0572) (5.8421, -60.3854) (6.425, -60.3854) knots 0 0 0 1 2 2 2
  spline S167 degree 2 poles (6.425, -60.3854) (6.9511, -60.3854) (7.4846, -60.9559) (7.4846, -61.4845) knots 0 0 0 1 2 2 2
  line L200 (7.4846, -61.4845) -> (7.4846, -61.7439)
  line L201 (7.4846, -61.7439) -> (5.9112, -61.7439)
  spline S168 degree 2 poles (5.9112, -61.7439) (5.9211, -61.9044) (6.0372, -62.1168) (6.1311, -62.1811) knots 0 0 0 1 2 2 2
  spline S169 degree 2 poles (6.1311, -62.1811) (6.2225, -62.2453) (6.4695, -62.2996) (6.6152, -62.2996) knots 0 0 0 1 2 2 2
  spline S170 degree 2 poles (6.6152, -62.2996) (6.7387, -62.2996) (6.9807, -62.2453) (7.082, -62.1984) knots 0 0 0 1 2 2 2
  spline S171 degree 2 poles (7.082, -62.1984) (7.1709, -62.1613) (7.3191, -62.0699) (7.3661, -62.0353) knots 0 0 0 1 2 2 2
  line L202 (7.3661, -62.0353) -> (7.4426, -62.0353)
  line L203 (7.4426, -62.0353) -> (7.4426, -62.6281)
  spline S172 degree 2 poles (7.4426, -62.6281) (7.3537, -62.6627) (7.2105, -62.722) (7.082, -62.7516) knots 0 0 0 1 2 2 2
  spline S173 degree 2 poles (7.082, -62.7516) (6.9659, -62.7837) (6.7189, -62.8183) (6.5411, -62.8183) knots 0 0 0 1 2 2 2
  spline S174 degree 2 poles (6.7782, -61.3116) (6.7733, -61.0844) (6.5732, -60.8448) (6.3682, -60.8448) knots 0 0 0 1 2 2 2
  spline S175 degree 2 poles (6.3682, -60.8448) (6.1582, -60.8448) (5.9211, -61.0967) (5.9088, -61.3116) knots 0 0 0 1 2 2 2
  line L204 (5.9088, -61.3116) -> (6.7782, -61.3116)
  line L205 (-7.7047, -67.775) -> (-8.6359, -67.775)
  line L206 (-8.6359, -67.775) -> (-9.4831, -66.6561)
  line L207 (-9.4831, -66.6561) -> (-9.7598, -66.6561)
  line L208 (-9.7598, -66.6561) -> (-9.7598, -67.775)
  line L209 (-9.7598, -67.775) -> (-10.5206, -67.775)
  line L210 (-10.5206, -67.775) -> (-10.5206, -64.727)
  line L211 (-10.5206, -64.727) -> (-9.2954, -64.727)
  spline S176 degree 2 poles (-9.2954, -64.727) (-9.041, -64.727) (-8.6656, -64.7912) (-8.505, -64.89) knots 0 0 0 1 2 2 2
  spline S177 degree 2 poles (-8.505, -64.89) (-8.342, -64.9938) (-8.1493, -65.3174) (-8.1493, -65.5644) knots 0 0 0 1 2 2 2
  spline S178 degree 2 poles (-8.1493, -65.5644) (-8.1493, -65.9126) (-8.4655, -66.3498) (-8.7298, -66.4783) knots 0 0 0 1 2 2 2
  line L212 (-8.7298, -66.4783) -> (-7.7047, -67.775)
  spline S179 degree 2 poles (-8.9348, -65.6607) (-8.9348, -65.5446) (-9.0237, -65.3791) (-9.125, -65.3347) knots 0 0 0 1 2 2 2
  spline S180 degree 2 poles (-9.125, -65.3347) (-9.1966, -65.305) (-9.372, -65.2877) (-9.5029, -65.2877) knots 0 0 0 1 2 2 2
  line L213 (-9.5029, -65.2877) -> (-9.7598, -65.2877)
  line L214 (-9.7598, -65.2877) -> (-9.7598, -66.1078)
  line L215 (-9.7598, -66.1078) -> (-9.54, -66.1078)
  spline S181 degree 2 poles (-9.54, -66.1078) (-9.3819, -66.1078) (-9.1571, -66.0682) (-9.0805, -66.0065) knots 0 0 0 1 2 2 2
  spline S182 degree 2 poles (-9.0805, -66.0065) (-9.0064, -65.9472) (-8.9348, -65.7891) (-8.9348, -65.6607) knots 0 0 0 1 2 2 2
  spline S183 degree 2 poles (-6.3413, -67.8368) (-6.9934, -67.8368) (-7.6874, -67.2143) (-7.6874, -66.6388) knots 0 0 0 1 2 2 2
  spline S184 degree 2 poles (-7.6874, -66.6388) (-7.6874, -66.0757) (-7.0403, -65.4038) (-6.4574, -65.4038) knots 0 0 0 1 2 2 2
  spline S185 degree 2 poles (-6.4574, -65.4038) (-5.9313, -65.4038) (-5.3977, -65.9744) (-5.3977, -66.503) knots 0 0 0 1 2 2 2
  line L216 (-5.3977, -66.503) -> (-5.3977, -66.7623)
  line L217 (-5.3977, -66.7623) -> (-6.9711, -66.7623)
  spline S186 degree 2 poles (-6.9711, -66.7623) (-6.9613, -66.9229) (-6.8452, -67.1353) (-6.7513, -67.1995) knots 0 0 0 1 2 2 2
  spline S187 degree 2 poles (-6.7513, -67.1995) (-6.6599, -67.2637) (-6.4129, -67.3181) (-6.2672, -67.3181) knots 0 0 0 1 2 2 2
  spline S188 degree 2 poles (-6.2672, -67.3181) (-6.1437, -67.3181) (-5.9016, -67.2637) (-5.8003, -67.2168) knots 0 0 0 1 2 2 2
  spline S189 degree 2 poles (-5.8003, -67.2168) (-5.7114, -67.1798) (-5.5632, -67.0884) (-5.5163, -67.0538) knots 0 0 0 1 2 2 2
  line L218 (-5.5163, -67.0538) -> (-5.4397, -67.0538)
  line L219 (-5.4397, -67.0538) -> (-5.4397, -67.6466)
  spline S190 degree 2 poles (-5.4397, -67.6466) (-5.5286, -67.6812) (-5.6719, -67.7404) (-5.8003, -67.7701) knots 0 0 0 1 2 2 2
  spline S191 degree 2 poles (-5.8003, -67.7701) (-5.9164, -67.8022) (-6.1634, -67.8368) (-6.3413, -67.8368) knots 0 0 0 1 2 2 2
  spline S192 degree 2 poles (-6.1042, -66.3301) (-6.1091, -66.1028) (-6.3092, -65.8632) (-6.5142, -65.8632) knots 0 0 0 1 2 2 2
  spline S193 degree 2 poles (-6.5142, -65.8632) (-6.7241, -65.8632) (-6.9613, -66.1152) (-6.9736, -66.3301) knots 0 0 0 1 2 2 2
  line L220 (-6.9736, -66.3301) -> (-6.1042, -66.3301)
  spline S194 degree 2 poles (-2.9401, -67.5107) (-2.9401, -67.8294) (-3.1253, -68.2764) (-3.2834, -68.3999) knots 0 0 0 1 2 2 2
  spline S195 degree 2 poles (-3.2834, -68.3999) (-3.444, -68.5259) (-3.8886, -68.6395) (-4.1603, -68.6395) knots 0 0 0 1 2 2 2
  spline S196 degree 2 poles (-4.1603, -68.6395) (-4.39, -68.6395) (-4.8025, -68.5803) (-4.9531, -68.5407) knots 0 0 0 1 2 2 2
  line L221 (-4.9531, -68.5407) -> (-4.9531, -67.9652)
  line L222 (-4.9531, -67.9652) -> (-4.8692, -67.9652)
  spline S197 degree 2 poles (-4.8692, -67.9652) (-4.8173, -67.985) (-4.6716, -68.0344) (-4.5975, -68.0541) knots 0 0 0 1 2 2 2
  spline S198 degree 2 poles (-4.5975, -68.0541) (-4.5085, -68.0764) (-4.3406, -68.106) (-4.2541, -68.106) knots 0 0 0 1 2 2 2
  spline S199 degree 2 poles (-4.2541, -68.106) (-4.0713, -68.106) (-3.8293, -68.0319) (-3.7675, -67.9627) knots 0 0 0 1 2 2 2
  spline S200 degree 2 poles (-3.7675, -67.9627) (-3.7058, -67.8911) (-3.6564, -67.6985) (-3.6564, -67.5503) knots 0 0 0 1 2 2 2
  line L223 (-3.6564, -67.5503) -> (-3.6564, -67.5083)
  spline S201 degree 2 poles (-3.6564, -67.5083) (-3.7774, -67.6145) (-4.0936, -67.7429) (-4.2615, -67.7429) knots 0 0 0 1 2 2 2
  spline S202 degree 2 poles (-4.2615, -67.7429) (-4.7086, -67.7429) (-5.1927, -67.1625) (-5.1927, -66.5672) knots 0 0 0 1 2 2 2
  spline S203 degree 2 poles (-5.1927, -66.5672) (-5.1927, -66.298) (-5.0445, -65.8682) (-4.9111, -65.7175) knots 0 0 0 1 2 2 2
  spline S204 degree 2 poles (-4.9111, -65.7175) (-4.7827, -65.5718) (-4.4246, -65.4137) (-4.2294, -65.4137) knots 0 0 0 1 2 2 2
  spline S205 degree 2 poles (-4.2294, -65.4137) (-4.054, -65.4137) (-3.7749, -65.5026) (-3.6613, -65.5767) knots 0 0 0 1 2 2 2
  line L224 (-3.6613, -65.5767) -> (-3.6341, -65.4754)
  line L225 (-3.6341, -65.4754) -> (-2.9401, -65.4754)
  line L226 (-2.9401, -65.4754) -> (-2.9401, -67.5107)
  line L227 (-3.6564, -67.0513) -> (-3.6564, -66.009)
  spline S206 degree 2 poles (-3.6564, -66.009) (-3.7082, -65.9843) (-3.8639, -65.9522) (-3.9429, -65.9522) knots 0 0 0 1 2 2 2
  spline S207 degree 2 poles (-3.9429, -65.9522) (-4.1998, -65.9522) (-4.4591, -66.2856) (-4.4591, -66.5845) knots 0 0 0 1 2 2 2
  spline S208 degree 2 poles (-4.4591, -66.5845) (-4.4591, -66.7327) (-4.4196, -66.9402) (-4.3677, -67.0192) knots 0 0 0 1 2 2 2
  spline S209 degree 2 poles (-4.3677, -67.0192) (-4.3159, -67.0982) (-4.1504, -67.1773) (-4.0219, -67.1773) knots 0 0 0 1 2 2 2
  spline S210 degree 2 poles (-4.0219, -67.1773) (-3.9256, -67.1773) (-3.7404, -67.1106) (-3.6564, -67.0513) knots 0 0 0 1 2 2 2
  line L228 (-0.2576, -67.775) -> (-0.9739, -67.775)
  line L229 (-0.9739, -67.775) -> (-0.9739, -67.5206)
  spline S211 degree 2 poles (-0.9739, -67.5206) (-1.1592, -67.6762) (-1.4704, -67.8392) (-1.6853, -67.8392) knots 0 0 0 1 2 2 2
  spline S212 degree 2 poles (-1.6853, -67.8392) (-2.0262, -67.8392) (-2.409, -67.407) (-2.409, -66.9723) knots 0 0 0 1 2 2 2
  line L230 (-2.409, -66.9723) -> (-2.409, -65.4754)
  line L231 (-2.409, -65.4754) -> (-1.6878, -65.4754)
  line L232 (-1.6878, -65.4754) -> (-1.6878, -66.6166)
  spline S213 degree 2 poles (-1.6878, -66.6166) (-1.6878, -66.7944) (-1.6705, -67.0217) (-1.6359, -67.0982) knots 0 0 0 1 2 2 2
  spline S214 degree 2 poles (-1.6359, -67.0982) (-1.6013, -67.1699) (-1.4655, -67.244) (-1.342, -67.244) knots 0 0 0 1 2 2 2
  spline S215 degree 2 poles (-1.342, -67.244) (-1.2679, -67.244) (-1.0604, -67.1699) (-0.9739, -67.1057) knots 0 0 0 1 2 2 2
  line L233 (-0.9739, -67.1057) -> (-0.9739, -65.4754)
  line L234 (-0.9739, -65.4754) -> (-0.2576, -65.4754)
  line L235 (-0.2576, -65.4754) -> (-0.2576, -67.775)
  line L236 (1.007, -67.775) -> (0.2907, -67.775)
  line L237 (0.2907, -67.775) -> (0.2907, -64.5912)
  line L238 (0.2907, -64.5912) -> (1.007, -64.5912)
  line L239 (1.007, -64.5912) -> (1.007, -67.775)
  spline S216 degree 2 poles (2.8225, -67.5305) (2.7484, -67.5922) (2.6323, -67.691) (2.5335, -67.7404) knots 0 0 0 1 2 2 2
  spline S217 degree 2 poles (2.5335, -67.7404) (2.4372, -67.7874) (2.2544, -67.8368) (2.0914, -67.8368) knots 0 0 0 1 2 2 2
  spline S218 degree 2 poles (2.0914, -67.8368) (1.7851, -67.8368) (1.3825, -67.4268) (1.3825, -67.1155) knots 0 0 0 1 2 2 2
  spline S219 degree 2 poles (1.3825, -67.1155) (1.3825, -66.8611) (1.5875, -66.545) (1.7801, -66.4536) knots 0 0 0 1 2 2 2
  spline S220 degree 2 poles (1.7801, -66.4536) (1.9753, -66.3597) (2.5162, -66.2856) (2.8274, -66.2658) knots 0 0 0 1 2 2 2
  line L240 (2.8274, -66.2658) -> (2.8274, -66.2535)
  spline S221 degree 2 poles (2.8274, -66.2535) (2.8274, -66.0633) (2.5458, -65.9176) (2.2643, -65.9176) knots 0 0 0 1 2 2 2
  spline S222 degree 2 poles (2.2643, -65.9176) (2.1383, -65.9176) (1.7974, -66.009) (1.6369, -66.0806) knots 0 0 0 1 2 2 2
  line L241 (1.6369, -66.0806) -> (1.5751, -66.0806)
  line L242 (1.5751, -66.0806) -> (1.5751, -65.5248)
  spline S223 degree 2 poles (1.5751, -65.5248) (1.6813, -65.4952) (2.1556, -65.4112) (2.3976, -65.4112) knots 0 0 0 1 2 2 2
  spline S224 degree 2 poles (2.3976, -65.4112) (2.9904, -65.4112) (3.5338, -65.8064) (3.5338, -66.2115) knots 0 0 0 1 2 2 2
  line L243 (3.5338, -66.2115) -> (3.5338, -67.775)
  line L244 (3.5338, -67.775) -> (2.8225, -67.775)
  line L245 (2.8225, -67.775) -> (2.8225, -67.5305)
  line L246 (2.8225, -67.1748) -> (2.8225, -66.6981)
  spline S225 degree 2 poles (2.8225, -66.6981) (2.6397, -66.7154) (2.4149, -66.7426) (2.3062, -66.7821) knots 0 0 0 1 2 2 2
  spline S226 degree 2 poles (2.3062, -66.7821) (2.2099, -66.8142) (2.1062, -66.9476) (2.1062, -67.0563) knots 0 0 0 1 2 2 2
  spline S227 degree 2 poles (2.1062, -67.0563) (2.1062, -67.2168) (2.2815, -67.3378) (2.452, -67.3378) knots 0 0 0 1 2 2 2
  spline S228 degree 2 poles (2.452, -67.3378) (2.5458, -67.3378) (2.7434, -67.2514) (2.8225, -67.1748) knots 0 0 0 1 2 2 2
  spline S229 degree 2 poles (4.9442, -67.8195) (4.507, -67.8195) (4.1069, -67.4589) (4.1069, -67.0488) knots 0 0 0 1 2 2 2
  line L247 (4.1069, -67.0488) -> (4.1069, -65.9744)
  line L248 (4.1069, -65.9744) -> (3.8327, -65.9744)
  line L249 (3.8327, -65.9744) -> (3.8327, -65.4754)
  line L250 (3.8327, -65.4754) -> (4.1069, -65.4754)
  line L251 (4.1069, -65.4754) -> (4.1069, -64.8184)
  line L252 (4.1069, -64.8184) -> (4.8232, -64.8184)
  line L253 (4.8232, -64.8184) -> (4.8232, -65.4754)
  line L254 (4.8232, -65.4754) -> (5.5148, -65.4754)
  line L255 (5.5148, -65.4754) -> (5.5148, -65.9744)
  line L256 (5.5148, -65.9744) -> (4.8232, -65.9744)
  line L257 (4.8232, -65.9744) -> (4.8232, -66.792)
  spline S230 degree 2 poles (4.8232, -66.792) (4.8232, -66.913) (4.8281, -67.0933) (4.8578, -67.1649) knots 0 0 0 1 2 2 2
  spline S231 degree 2 poles (4.8578, -67.1649) (4.8874, -67.2366) (5.0331, -67.3205) (5.1715, -67.3205) knots 0 0 0 1 2 2 2
  spline S232 degree 2 poles (5.1715, -67.3205) (5.2307, -67.3205) (5.416, -67.2711) (5.453, -67.2514) knots 0 0 0 1 2 2 2
  line L258 (5.453, -67.2514) -> (5.5148, -67.2514)
  line L259 (5.5148, -67.2514) -> (5.5148, -67.7553)
  spline S233 degree 2 poles (5.5148, -67.7553) (5.3987, -67.7849) (5.1369, -67.8195) (4.9442, -67.8195) knots 0 0 0 1 2 2 2
  spline S234 degree 2 poles (8.012, -66.6265) (8.012, -67.1946) (7.392, -67.8467) (6.8264, -67.8467) knots 0 0 0 1 2 2 2
  spline S235 degree 2 poles (6.8264, -67.8467) (6.2632, -67.8467) (5.6383, -67.1946) (5.6383, -66.6265) knots 0 0 0 1 2 2 2
  spline S236 degree 2 poles (5.6383, -66.6265) (5.6383, -66.0534) (6.2632, -65.4038) (6.8264, -65.4038) knots 0 0 0 1 2 2 2
  spline S237 degree 2 poles (6.8264, -65.4038) (7.3895, -65.4038) (8.012, -66.0559) (8.012, -66.6265) knots 0 0 0 1 2 2 2
  spline S238 degree 2 poles (7.2784, -66.6314) (7.2784, -66.4264) (7.2117, -66.1522) (7.1524, -66.0707) knots 0 0 0 1 2 2 2
  spline S239 degree 2 poles (7.1524, -66.0707) (7.0882, -65.9843) (6.9276, -65.9176) (6.8264, -65.9176) knots 0 0 0 1 2 2 2
  spline S240 degree 2 poles (6.8264, -65.9176) (6.7276, -65.9176) (6.572, -65.9769) (6.5077, -66.0608) knots 0 0 0 1 2 2 2
  spline S241 degree 2 poles (6.5077, -66.0608) (6.446, -66.1399) (6.3719, -66.419) (6.3719, -66.6314) knots 0 0 0 1 2 2 2
  spline S242 degree 2 poles (6.3719, -66.6314) (6.3719, -66.8414) (6.4411, -67.1007) (6.4979, -67.1798) knots 0 0 0 1 2 2 2
  spline S243 degree 2 poles (6.4979, -67.1798) (6.5547, -67.2588) (6.7276, -67.3329) (6.8313, -67.3329) knots 0 0 0 1 2 2 2
  spline S244 degree 2 poles (6.8313, -67.3329) (6.9178, -67.3329) (7.0956, -67.2588) (7.1499, -67.1847) knots 0 0 0 1 2 2 2
  spline S245 degree 2 poles (7.1499, -67.1847) (7.2117, -67.0982) (7.2784, -66.8488) (7.2784, -66.6314) knots 0 0 0 1 2 2 2
  line L260 (9.9361, -66.1547) -> (9.8768, -66.1547)
  spline S246 degree 2 poles (9.8768, -66.1547) (9.8349, -66.1399) (9.6792, -66.1251) (9.5854, -66.1251) knots 0 0 0 1 2 2 2
  spline S247 degree 2 poles (9.5854, -66.1251) (9.4742, -66.1251) (9.2248, -66.1917) (9.1087, -66.2362) knots 0 0 0 1 2 2 2
  line L261 (9.1087, -66.2362) -> (9.1087, -67.775)
  line L262 (9.1087, -67.775) -> (8.3924, -67.775)
  line L263 (8.3924, -67.775) -> (8.3924, -65.4754)
  line L264 (8.3924, -65.4754) -> (9.1087, -65.4754)
  line L265 (9.1087, -65.4754) -> (9.1087, -65.8064)
  spline S248 degree 2 poles (9.1087, -65.8064) (9.1581, -65.762) (9.331, -65.6236) (9.4026, -65.5817) knots 0 0 0 1 2 2 2
  spline S249 degree 2 poles (9.4026, -65.5817) (9.4816, -65.5347) (9.6891, -65.468) (9.7805, -65.468) knots 0 0 0 1 2 2 2
  spline S250 degree 2 poles (9.7805, -65.468) (9.8151, -65.468) (9.9015, -65.473) (9.9361, -65.4754) knots 0 0 0 1 2 2 2
  line L266 (9.9361, -65.4754) -> (9.9361, -66.1547)
  spline S251 degree 2 poles (-76.2156, 3.9591) (-76.2156, 3.5713) (-76.3959, 2.9241) (-76.5861, 2.692) knots 0 0 0 1 2 2 2
  spline S252 degree 2 poles (-76.5861, 2.692) (-76.7837, 2.4573) (-77.3666, 2.2054) (-77.7914, 2.2054) knots 0 0 0 1 2 2 2
  spline S253 degree 2 poles (-77.7914, 2.2054) (-77.9347, 2.2054) (-78.2459, 2.2424) (-78.2978, 2.2572) knots 0 0 0 1 2 2 2
  line L267 (-78.2978, 2.2572) -> (-78.2978, 2.855)
  line L268 (-78.2978, 2.855) -> (-78.2385, 2.855)
  spline S254 degree 2 poles (-78.2385, 2.855) (-78.1817, 2.8253) (-77.9693, 2.7611) (-77.784, 2.7611) knots 0 0 0 1 2 2 2
  spline S255 degree 2 poles (-77.784, 2.7611) (-77.6334, 2.7611) (-77.3543, 2.8402) (-77.2555, 2.9266) knots 0 0 0 1 2 2 2
  spline S256 degree 2 poles (-77.2555, 2.9266) (-77.1492, 3.018) (-77.0109, 3.2872) (-76.9862, 3.4898) knots 0 0 0 1 2 2 2
  spline S257 degree 2 poles (-76.9862, 3.4898) (-77.1492, 3.3885) (-77.4308, 3.2798) (-77.6408, 3.2798) knots 0 0 0 1 2 2 2
  spline S258 degree 2 poles (-77.6408, 3.2798) (-77.7964, 3.2798) (-78.0854, 3.3638) (-78.2039, 3.4527) knots 0 0 0 1 2 2 2